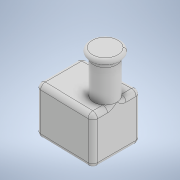
# Autodesk Inventor part: vagonetka
Saved by Autodesk Inventor 2020 (Build 240168000, 168)
## iProperties
Created: 2022-07-29
Part Number: vagonetka
Material: Типовые
Document SubType Name: Modeling
Designer: akapu
Density: 1 g/cm^3
Appearance: По умолчанию
Author: akapu
Autodesk Inventor part; units mm, degrees
ref_plane "YZ Plane" through (0, 0, 0) normal (1, 0, 0) x (0, 1, 0)
ref_plane "XZ Plane" through (0, 0, 0) normal (0, 1, 0) x (-1, 0, 0)
ref_plane "XY Plane" through (0, 0, 0) normal (0, 0, 1) x (1, 0, 0)
sketch "Эскиз2" plane through (0, 0, 0) normal (0, 1, 0) x (-1, 0, 0)
  line L0 (-12, 0) -> (-12, 5.2)
  line L1 (-12, 0) -> (-12, -5.2)
  line L2 (-12, 0) -> (0.5, 0)
  line L3 (0.5, 0) -> (0.5, 4.9)
  line L4 (0.5, 4.9) -> (-12, 5.2)
  line L5 (0.5, 0) -> (0.5, -4.9)
  line L6 (0.5, -4.9) -> (-12, -5.2)
  point P0 (0, 0)
  dimension "d3" = 5.2
  dimension "d4" = 5.2
  dimension "d20" = 12.5
  dimension "d21" = 4.9
  dimension "d22" = 4.9
  constraints: 14 end point, 2 point on line, 2 vertical, 1 horizontal
  measures "d3" distance of L0.start L0.end
  measures "d4" distance of L0.start L1.end
  measures "d20" distance of L0.start L2.end
  measures "d21" distance of L2.end L3.end
  measures "d22" distance of L2.end L5.end
extrude "Выдавливание1" add sketch "Эскиз2" along normal blind 10.2
sketch "Эскиз3" plane through (0, 10.2, 0) normal (0, 1, 0) x (1, 0, 0)
  line L0 (12, -4.1832) -> (12, 4.1832) projected
  line L1 (12, 0) -> (7, 0)
  circle A0 centre (9.5, 0) radius 2.5
  point P0 (0, 0)
  dimension "d8" = 5
  constraints: 2 end point, 2 midpoint, 1 horizontal, 1 horizontal alignment, 2 other
  measures "d8" distance of L1.start L1.end
extrude "Выдавливание2" add sketch "Эскиз3" along normal blind 7
sketch "Эскиз4" plane through (9.5, 17.2, 0) normal (0, 1, 0) x (1, 0, 0)
  circle A0 centre (0, 0) radius 3.5
  point P0 (-9.5, 0)
  dimension "d11" = 7
  constraints: 1 centre point
  measures "d11" diameter of A0
extrude "Выдавливание3" add sketch "Эскиз4" along normal blind 2
fillet "Сопряжение2" radius 1 1 edges at (6, 17.2, 0) inverted yes
fillet "Сопряжение3" radius 0.6 2 edges at (6, 19.2, 0) (6, 18.2, 0)
fillet "Сопряжение6" radius 1 13 edges at (5.75, 10.2, -5.05) (-0.5, 5.1, -4.9) (-0.5, 0, 0) (-0.5, 5.1, 4.9) (-0.5, 10.2, 0) (5.75, 0, -5.05) (5.75, 0, 5.05) (12, 0, 0) (12, 5.1, 5.2) (5.75, 10.2, 5.05) (12, 10.2, 2.6) (12, 10.2, -2.6) (12, 5.1, -5.2)
